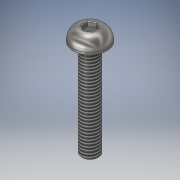
# Autodesk Inventor part: Wheel coupler screw
Saved by Autodesk Inventor 2018 (Build 220112000, 112)
## iProperties
Created: 2018-05-02
Part Number: Wheel coupler screw
Material: Stainless Steel
Document SubType Name: Modeling
Designer: Ajith Thomas
Mass: 3.23612 g
Surface Area: 4.41521 cm^2
Volume: 0.404515 cm^3
Density: 8 g/cm^3
Appearance: Semi-Polished
Author: Ajith Thomas
Autodesk Inventor part; units mm, degrees
ref_plane "YZ Plane" through (0, 0, 0) normal (1, 0, 0) x (0, 1, 0)
ref_plane "XZ Plane" through (0, 0, 0) normal (0, 1, 0) x (-1, 0, 0)
ref_plane "XY Plane" through (0, 0, 0) normal (0, 0, 1) x (1, 0, 0)
sketch "Sketch1" plane through (0, 0, 0) normal (0, 1, 0) x (-1, 0, 0)
  circle A0 centre (0, 0) radius 4
  dimension "d0" = 8
  constraints: 1 centre point, 1 coincident
  measures "d0" diameter of A0
extrude "Extrusion1" add sketch "Sketch1" along normal blind 3
fillet "Fillet1" radius 2.5 1 edges at (4, 3, 0)
sketch "Sketch2" plane through (0, 3, 0) normal (0, 1, 0) x (1, 0, 0)
  circle A0 centre (0, 0) radius 1.5 projected
  line L0 (0, 1.5) -> (1.299, 0.75)
  line L1 (1.299, 0.75) -> (1.299, -0.75)
  line L2 (1.299, -0.75) -> (0, -1.5)
  line L3 (0, -1.5) -> (-1.299, -0.75)
  line L4 (-1.299, -0.75) -> (-1.299, 0.75)
  line L5 (-1.299, 0.75) -> (0, 1.5)
  constraints: 12 end point, 1 coincident, 1 vertical alignment, 14 other
extrude "Extrusion2" cut sketch "Sketch2" against normal blind 1 contours L1 L2 L3 L4 L5 L0
fillet "Fillet2" radius 0.2 6 edges at (-0.6495, 3, 1.125) (-1.299, 3, 0) (-0.6495, 3, -1.125) (0.6495, 3, -1.125) (1.299, 3, 0) (0.6495, 3, 1.125)
sketch "Sketch3" plane through (0, 0, 0) normal (0, -1, 0) x (1, 0, 0)
  circle A0 centre (0, 0) radius 4 construction
  circle A1 centre (0, 0) radius 2
  dimension "d7" = 4
  constraints: 1 centre point, 1 coincident
  measures "d7" diameter of A1
extrude "Extrusion3" add sketch "Sketch3" along normal blind 23
chamfer "Chamfer1" distance 0.25 angle 45 1 edges at (-2, -23, 0)
thread "Thread1" size "M4x0.7" class "6g" standard "ANSI Metric M Profile" full length
body "Solid1"
